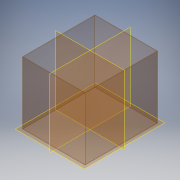
# Autodesk Inventor part: AM14U3-gameVolume
Saved by Autodesk Inventor 2018.2 (Build 222227000, 227)
## iProperties
Created: 2018-01-09
Part Number: AM14U3-gameVolume
Material: Polycarbonate, Smoke
Document SubType Name: Modeling
Designer: steele
Density: 1.2 g/cm^3
Appearance: Polycarbonate - Smoked
Author: steele
Autodesk Inventor part; units mm, degrees
sketch "Sketch1" plane through (0, 0, 0) normal (0, 1, 0) x (-1, 0, 0)
  line L0 (704.85, 816.737) -> (-704.85, 816.737)
  line L1 (-704.85, 816.737) -> (-704.85, -816.737)
  line L2 (-704.85, -816.737) -> (704.85, -816.737)
  line L3 (704.85, -816.737) -> (704.85, 816.737)
  line L4 (704.85, 816.737) -> (-704.85, -816.737) construction
  line L5 (-704.85, 816.737) -> (704.85, -816.737) construction
  line L6 (692.15, 804.037) -> (-692.15, 804.037)
  line L7 (-692.15, 804.037) -> (-692.15, -804.037)
  line L8 (-692.15, -804.037) -> (692.15, -804.037)
  line L9 (692.15, -804.037) -> (692.15, 804.037)
  line L10 (692.15, 804.037) -> (-692.15, -804.037) construction
  line L11 (-692.15, 804.037) -> (692.15, -804.037) construction
  point P0 (0, 0)
  dimension "d0" = 1409.7
  dimension "d1" = 1633.474
  dimension "d2" = 12.7
  dimension "d3" = 12.7
  constraints: 24 end point, 5 parallel, 4 midpoint, 2 perpendicular, 1 horizontal
  measures "d0" distance of L0.start L0.end
  measures "d1" distance of L1.end L0.end
  measures "d2" distance between parallel lines of L1 L7
  measures "d3" distance between parallel lines of L0 L6
extrude "Extrusion1" add sketch "Sketch1" along normal blind 1397
body "Solid1"
